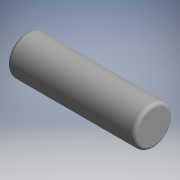
# Autodesk Inventor part: HK0709FMRO
Saved by Autodesk Inventor 2017.3 (Build 213256000, 256)
## iProperties
Part Number: HK0709FMRO
Material: Generic
Catalog Web Link: www.cadenas.de
Description: Needle Roller Shell Bearings open-ended RO-
Vendor: NTN
Document SubType Name: Modeling
Designer: partserver
Manufacturer: NTN
Mass: 0.0088012 g
Surface Area: 0.265411 cm^2
Volume: 0.0088012 cm^3
Density: 1 g/cm^3
Appearance: PSOLRGB-192-192-192
Category: PARTsolutions
Company: NTN
Title: HK0709FMRO
Author: Cadenas PARTsolutions
PSOL_IDENT_0: {$CADENAS_DATA\23d-libs\ntn\needle_roler_bearings\needle_roller_shell_bearings_open_ended_ro.prj},19
PSOL_IDENT_1: 6 {VTYP=3D},{NB=HK0709FMRO},{LINA=HK0709FMRO},{NN=Needle Roller Shell Bearings open-ended RO},{DATE=
PSOL_IDENT_2: 26.11.2019 01:59:50},{GEOMDATE=26.11.2019 00:10:00},{VERSION=},{LINEID=50},{WBVAR=},{WBNUMERIC=}  {N
PSOL_IDENT_3: B=HK0709FMRO},{LINA=HK0709FMRO},{KT=DUMMY},{FW=7},{D=11.0},{C=9},{ORDER=HK0709FM},{CR=3150},{COR=293
PSOL_IDENT_4: 0},{CRF=320},{CORF=299},{LSG=23000},{LSO=34000},{MASS=0.0025},{IT=-},{RT=1.6},{VER=1},{T=0.500},{DW=
PSOL_IDENT_5: 1.500},{LW=5.000},{NR=10.000},{CID=7.750},{CD=9.250},{CW=7.600},{SD=7.350}
NB: HK0709FMRO
NN: Needle Roller Shell Bearings open-ended RO
NBSYN: $ORDER.RO
LINA: HK0709FMRO
CATALOG: NTN Corporation
FW: 7
D: 11
C: 9
ORDER: HK0709FM
CR: 3150
COR: 2930
CRF: 320
CORF: 299
LSG: 23000
LSO: 34000
MASS: 0.0025
IT: -
RT: 1.6
VER: 1
SUPPLIER: NTN
ARTICLENO: HK0709FMRO
BOMINFO: HK0709FMRO
CREATOR: CADENAS GmbH
Autodesk Inventor part; units mm, degrees
ref_plane "YZ Plane" through (0, 0, 0) normal (1, 0, 0) x (0, 1, 0)
ref_plane "XZ Plane" through (0, 0, 0) normal (0, 1, 0) x (-1, 0, 0)
ref_plane "XY Plane" through (0, 0, 0) normal (0, 0, 1) x (1, 0, 0)
sketch "Sketch_1" plane through (0, 0, 0) normal (0, 0, 1) x (1, 0, 0)
  line L0 (2.5, 0) -> (-2.5, 0)
  line L1 (-2.5, 0) -> (-2.5, 0.6167)
  arc A0 (-2.3667, 0.75) -> (-2.5, 0.6167) centre (-2.3667, 0.6167) ccw
  line L2 (-2.3667, 0.75) -> (2.3667, 0.75)
  arc A1 (2.5, 0.6167) -> (2.3667, 0.75) centre (2.3667, 0.6167) ccw
  line L3 (2.5, 0.6167) -> (2.5, 0)
  line L4 (2.5, 0) -> (-2.5, 0)
  constraints: 10 end point, 4 point on circle, 2 centre point
revolve "Revolution1" add sketch "Sketch_1" angle 360 about axis through (2.5, 0, 0) along (1, 0, 0)
ref_plane "IP_1_XY" through (0, 0, 0) normal (1, 0, 0) x (0, 0, -1)
ref_plane "IP_1_YZ" through (0, 0, 0) normal (0, 0, -1) x (0, 1, 0)
ref_plane "IP_1_ZX" through (0, 0, 0) normal (0, 1, 0) x (1, 0, 0)
body "Solid1"
